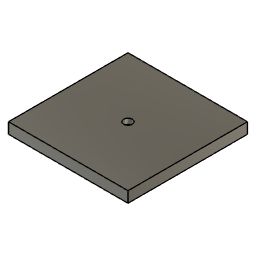
sand_cube_bot (Autodesk Fusion 360 design; units mm, degrees)
Autodesk Fusion 360 part; units mm, degrees
sketch "Sketch1" plane through (0, 0, 0) normal (0, 0, 1) x (1, 0, 0)
  line L0 (0, 0) -> (55, 0)
  line L1 (55, 0) -> (55, 55)
  line L2 (55, 55) -> (0, 55)
  line L3 (0, 55) -> (0, 0)
  dimension "d1" = 55
  dimension "d2" = 55
  constraint horizontal L0
  constraint vertical L1
  constraint horizontal L2
  constraint vertical L3
  constraint coincident L0.start L3.end
  measures "d1" distance of L0.start L0.end
  measures "d2" distance of L0.start L2.end
extrude "Extrude1" add sketch "Sketch1" along normal blind 5
sketch "Sketch2" plane through (0, 0, 5) normal (0, 0, 1) x (-1, 0, 0)
  line L0 (0, -55) -> (0, 0)
  line L1 (0, 0) -> (-55, 0)
  line L2 (-55, 0) -> (-55, -55)
  line L3 (-55, -55) -> (0, -55)
  circle A0 centre (-27.5, -27.5) radius 2
  dimension "d5" = 4
  measures "d5" diameter of A0
extrude "Extrude2" cut sketch "Sketch2" against normal blind 2.5 contours A0
